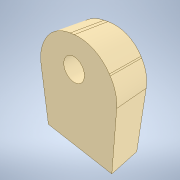
# Autodesk Inventor part: Крепление шкива
Saved by Autodesk Inventor 2021.1 (Build 251245010, 245A)
## iProperties
Created: 2026-04-16
Part Number: Крепление шкива
Material: Типовые
Document SubType Name: Modeling
Designer: Андрей Тарасов
Density: 1 g/cm^3
Appearance: По умолчанию
Author: Андрей Тарасов
Autodesk Inventor part; units mm, degrees
ref_plane "YZ Plane" through (0, 0, 0) normal (1, 0, 0) x (0, 1, 0)
ref_plane "XZ Plane" through (0, 0, 0) normal (0, 1, 0) x (-1, 0, 0)
ref_plane "XY Plane" through (0, 0, 0) normal (0, 0, 1) x (1, 0, 0)
sketch "Эскиз1" plane through (0, 0, 0) normal (0, 0, 1) x (1, 0, 0)
  circle A0 centre (0, 0) radius 2
  line L0 (-7.5, -14.5) -> (7.5, -14.5)
  line L1 (7.5, -14.5) -> (7.5, 0)
  line L2 (7.5, 0) -> (-7.5, 0) construction
  line L3 (-7.5, 0) -> (-7.5, -14.5)
  line L4 (0, -18.7) -> (0, 10.7) construction
  circle A1 centre (0, 0) radius 6.5 construction
  line L5 (-7.5, 0) -> (-4, 5)
  line L6 (-4, 5) -> (4, 5)
  line L7 (4, 5) -> (7.5, 0)
  point P0 (0, 5)
  point P1 (0, -14.5)
  dimension "d0" = 4
  dimension "d6" = 13
  dimension "d8" = 8
  dimension "d11" = 15
  dimension "d12" = 5
  dimension "d13" = 14.5
  constraints: 14 end point, 3 midpoint, 2 centre point, 2 coincident, 2 horizontal, 2 perpendicular, 2 point on line
  measures "d0" diameter of A0
  measures "d6" diameter of A1
  measures "d8" distance of L5.end L6.end
  measures "d11" distance between parallel lines of L1 L3
  measures "d12" distance between parallel lines of L6 L2
  measures "d13" distance between parallel lines of L0 L2
extrude "Выдавливание1" add sketch "Эскиз1" along normal blind 6
fillet "Сопряжение1" radius 7 4 edges at (-7.5, 0, 3) (-4, 5, 3) (4, 5, 3) (7.5, 0, 3)
